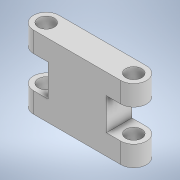
# Autodesk Inventor part: link_v4
Saved by Autodesk Inventor 2022 (Build 260153000, 153)
## iProperties
Created: 2022-06-04
Part Number: link_v4
Material: Generic
Document SubType Name: Modeling
Designer: kylem
Density: 1 g/cm^3
Appearance: Default
Author: kylem
Autodesk Inventor part; units mm, degrees
ref_plane "YZ Plane" through (0, 0, 0) normal (1, 0, 0) x (0, 1, 0)
ref_plane "XZ Plane" through (0, 0, 0) normal (0, 1, 0) x (-1, 0, 0)
ref_plane "XY Plane" through (0, 0, 0) normal (0, 0, 1) x (1, 0, 0)
sketch "Sketch1" plane through (0, 0, 0) normal (0, 1, 0) x (-1, 0, 0)
  line L0 (0, 0) -> (12, 0)
  circle A0 centre (12, 0) radius 1.1
  circle A1 centre (0, 0) radius 1.1
  circle A2 centre (12, 0) radius 1.75
  circle A3 centre (0, 0) radius 1.75
  line L1 (12, 1.75) -> (0, 1.75)
  line L2 (12, -1.75) -> (0, -1.75)
  dimension "d0" = 12
  dimension "d1" = 2.2
  dimension "d2" = 2.2
  dimension "d3" = 3.5
  dimension "d4" = 3.5
  constraints: 6 end point, 4 centre point, 4 coincident, 4 point on circle, 2 tangent, 1 horizontal
  measures "d0" distance of L0.start L0.end
  measures "d1" diameter of A0
  measures "d2" diameter of A1
  measures "d3" diameter of A2
  measures "d4" diameter of A3
extrude "Extrusion1" add sketch "Sketch1" along normal mid plane 10
sketch "Sketch2" plane through (0, 5, -1.75) normal (0, 0, -1) x (-1, 0, 0)
  line L0 (0, 0) -> (-1.75, 0) projected
  line L1 (0, 0) -> (2, 0)
  line L2 (0, 0) -> (12, 0) projected
  line L3 (13.75, 0) -> (12, 0) projected
  line L4 (12, -10) -> (0, -10) projected
  line L5 (12, 0) -> (10, 0)
  line L6 (10, 0) -> (10, -10)
  line L7 (10, -10) -> (12, -10)
  line L8 (12, -10) -> (12, 0)
  line L9 (2, 0) -> (0, 0)
  line L10 (0, 0) -> (0, -10)
  line L11 (0, -10) -> (2, -10)
  line L12 (2, -10) -> (2, 0)
  line L13 (10, -5) -> (10, -2.8)
  line L14 (10, -5) -> (10, -7.2)
  line L15 (10, -2.8) -> (14.3715, -2.8)
  line L16 (14.3715, -2.8) -> (14.3715, -7.2)
  line L17 (14.3715, -7.2) -> (10, -7.2)
  line L18 (10, -7.2) -> (10, -2.8)
  line L19 (2, -5) -> (2, -2.8)
  line L20 (2, -5) -> (2, -7.2)
  line L21 (2, -7.2) -> (-5.4326, -7.2)
  line L22 (-5.4326, -7.2) -> (-5.4326, -2.8)
  line L23 (-5.4326, -2.8) -> (2, -2.8)
  line L24 (2, -2.8) -> (2, -7.2)
  point P0 (0, -5)
  dimension "d7" = 2
  dimension "d8" = 2
  dimension "d9" = 2.2
  dimension "d10" = 2.2
  dimension "d11" = 2.2
  dimension "d12" = 2.2
  constraints: 42 end point, 8 parallel, 7 point on line, 4 horizontal, 4 perpendicular, 2 midpoint
  measures "d7" distance of L0.start L1.end
  measures "d8" distance of L7.end L6.end
  measures "d9" distance of L13.start L13.end
  measures "d10" distance of L13.start L14.end
  measures "d11" distance of L19.start L19.end
  measures "d12" distance of L19.start L20.end
extrude "Extrusion2" cut sketch "Sketch2" against normal blind 10 contours L23 L12 L21 L10 | L10 L21 L22 L23 | L15 L8 L17 L6 | L15 L16 L17 L8
body "Solid1"
